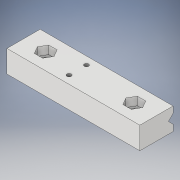
# Autodesk Inventor part: X-Axis_Mount_Slide_Endstop_MountLM3046
Saved by Autodesk Inventor 2020.3 (Build 243373000, 373)
## iProperties
Created: 2019-11-08
Part Number: X-Axis_Mount_Slide_Endstop_MountLM3046
Material: Acetal Resin, White
Document SubType Name: Modeling
Designer: Sarah Hall
Density: 1.425 g/cm^3
Appearance: Smooth - White
Author: Sarah Hall
Autodesk Inventor part; units mm, degrees
ref_plane "YZ Plane" through (0, 0, 0) normal (1, 0, 0) x (0, 1, 0)
ref_plane "XZ Plane" through (0, 0, 0) normal (0, 1, 0) x (-1, 0, 0)
ref_plane "XY Plane" through (0, 0, 0) normal (0, 0, 1) x (1, 0, 0)
sketch "Sketch1" plane through (0, 0, 0) normal (0, 1, 0) x (-1, 0, 0)
  line L0 (-38.1, 9.525) -> (38.1, 9.525)
  line L1 (38.1, 9.525) -> (38.1, -9.525)
  line L2 (38.1, -9.525) -> (-38.1, -9.525)
  line L3 (-38.1, -9.525) -> (-38.1, 9.525)
  line L4 (-38.1, 9.525) -> (38.1, -9.525) construction
  line L5 (38.1, 9.525) -> (-38.1, -9.525) construction
  point P0 (0, 0)
  dimension "d0" = 76.2
  dimension "d1" = 19.05
  constraints: 12 end point, 2 midpoint, 2 parallel, 1 horizontal, 1 perpendicular
  measures "d0" distance of L1.end L2.end
  measures "d1" distance of L0.end L1.end
extrude "Extrusion1" add sketch "Sketch1" along normal mid plane 12.7
sketch "Sketch2" plane through (38.1, -6.35, -9.525) normal (1, 0, 0) x (0, 0, -1)
  line L0 (0, 3.663) -> (-2.687, 6.35)
  line L1 (-2.687, 6.35) -> (0, 9.037)
  line L2 (0, 9.037) -> (2.687, 6.35)
  line L3 (2.687, 6.35) -> (0, 3.663)
  line L4 (-19.05, 12.7) -> (0, 12.7) projected
  line L5 (0, 12.7) -> (0, 0) projected
  point P0 (-9.525, 6.35)
  point P1 (0, 6.35)
  dimension "d4" = 45
  dimension "d5" = 3.8
  constraints: 8 end point, 2 parallel, 2 perpendicular, 1 horizontal alignment, 1 midpoint, 1 point on line
  measures "d4" angle of L4 L3
  measures "d5" distance of L0.end L1.end
extrude "Extrusion2" cut sketch "Sketch2" against normal through all
sketch "Sketch5" plane through (0, 6.35, 0) normal (0, 1, 0) x (1, 0, 0)
  line L0 (-38.1, 9.525) -> (-38.1, -9.525) projected
  line L1 (38.1, -9.525) -> (38.1, 9.525) projected
  point P0 (0, 0)
  point P1 (-25.4, 0)
  point P2 (25.4, 0)
  dimension "d18" = 12.7
  dimension "d19" = 12.7
  constraints: 2 horizontal alignment
  measures "d18" distance from line of L0 point (-25.4, 0)
  measures "d19" distance from line of L1 point (25.4, 0)
hole "Hole1" at (-25.4, 6.35, 0) at (25.4, 6.35, 0) direction (0, -1, 0) diameter 5.3086 end through all clearance for "Flat Head Machine Screw" size "M5" standard "Ansi Metric M Profile"
sketch "Sketch7" plane through (0, 6.35, 0) normal (0, 1, 0) x (1, 0, 0)
  circle A0 centre (-25.4, 0) radius 2.6543 projected
  circle A1 centre (25.4, 0) radius 2.6543 projected
  line L0 (-23.004, 4.15) -> (-20.608, 0)
  line L1 (-20.608, 0) -> (-23.004, -4.15)
  line L2 (-23.004, -4.15) -> (-27.796, -4.15)
  line L3 (-27.796, -4.15) -> (-30.192, 0)
  line L4 (-30.192, 0) -> (-27.796, 4.15)
  line L5 (-27.796, 4.15) -> (-23.004, 4.15)
  line L6 (23.004, -4.15) -> (20.608, 0)
  line L7 (20.608, 0) -> (23.004, 4.15)
  line L8 (23.004, 4.15) -> (27.796, 4.15)
  line L9 (27.796, 4.15) -> (30.192, 0)
  line L10 (30.192, 0) -> (27.796, -4.15)
  line L11 (27.796, -4.15) -> (23.004, -4.15)
  point P0 (0, 0)
  dimension "d39" = 8.3
  dimension "d40" = 8.3
  constraints: 24 end point, 2 coincident, 2 horizontal, 26 other
  measures "d39" distance between parallel lines of L5 L2
  measures "d40" distance between parallel lines of L8 L11
extrude "Extrusion5" cut sketch "Sketch7" against normal blind 4.7625 contours A1 | L0 L1 L2 L3 L4 L5 | L6 L7 L8 L9 L10 L11
sketch "Sketch8" plane through (0, 6.35, 0) normal (0, 1, 0) x (1, 0, 0)
  point P0 (0, 0)
  point P1 (-7, -5)
  point P2 (-7, 5)
  dimension "d43" = 10
  dimension "d52" = 7
  dimension "d53" = 5
  constraints: 1 vertical alignment
  measures "d43" distance of point (-7, -5) point (-7, 5)
  measures "d52" horizontal distance of point (0, 0) point (-7, 5)
  measures "d53" vertical distance of point (0, 0) point (-7, 5)
hole "Hole3" at (-7, 6.35, 5) at (-7, 6.35, -5) direction (0, -1, 0) diameter 2.459 depth 8.7884 thread size "M3x0.5" class "6H" standard "ANSI Metric M Profile"
equation "\"d40\" = d39"
body "Solid1"
